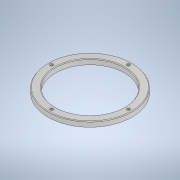
# Autodesk Inventor part: turntable_out_8_23
Saved by Autodesk Inventor 2022 (Build 260153070, 153G)
## iProperties
Created: 2021-08-23
Part Number: turntable_out_8_23
Material: アルミニウム 6061-AHC
Document SubType Name: Modeling
Designer: sky
Density: 2.7 g/cm^3
Appearance: アルミニウム - ダーク
Mass: 112.569 g
Surface Area: 168.607 cm^2
Volume: 41.6923 cm^3
Author: sky
Autodesk Inventor part; units mm, degrees
ref_plane "YZ Plane" through (0, 0, 0) normal (1, 0, 0) x (0, 1, 0)
ref_plane "XZ Plane" through (0, 0, 0) normal (0, 1, 0) x (-1, 0, 0)
ref_plane "XY Plane" through (0, 0, 0) normal (0, 0, 1) x (1, 0, 0)
sketch "スケッチ1" plane through (0, 0, 0) normal (0, 1, 0) x (-1, 0, 0)
  circle A0 centre (0, 0) radius 57.5
  circle A1 centre (0, 0) radius 70
  dimension "d0" = 115
  dimension "d1" = 140
  constraints: 2 centre point, 2 coincident
  measures "d0" diameter of A0
  measures "d1" diameter of A1
extrude "押し出し1" add sketch "スケッチ1" along normal blind 8.5
fillet "フィレット1" radius 1 2 edges at (57.5, 8.5, 0) (70, 8.5, 0)
sketch "スケッチ3" plane through (0, 8.5, 0) normal (0, 1, 0) x (1, 0, 0)
  circle A0 centre (0, 0) radius 64
  point P0 (0, 64)
  point P1 (64, 0)
  point P2 (0, -64)
  point P3 (-64, 0)
  dimension "d19" = 128
  constraints: 4 point on circle, 1 centre point, 1 coincident
  measures "d19" diameter of A0
hole "穴2" at (0, 8.5, -64) at (64, 8.5, 0) at (0, 8.5, 64) at (-64, 8.5, 0) direction (0, -1, 0) diameter 5.1 end through all
